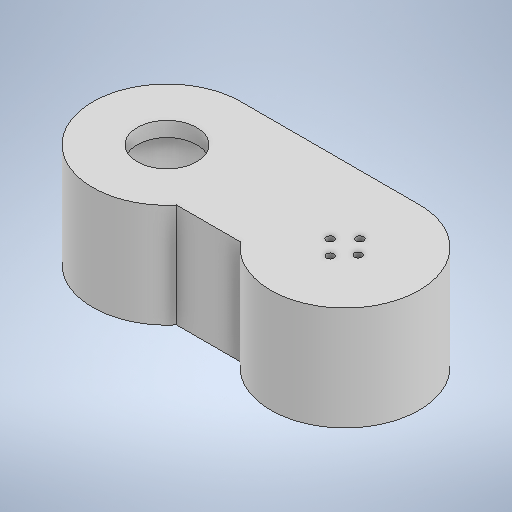
# Autodesk Inventor part: con_v6_d1
Saved by Autodesk Inventor 2025.4 (Build 294407000, 407)
## iProperties
Created: 2026-07-20
Part Number: con_v6_d1
Material: Generic
Document SubType Name: Modeling
Designer: Franchesca
Density: 1 g/cm^3
Appearance: Default
Author: Franchesca
## iProperties of the stored document con_v6_d1_3DPrint.ipt
Created: 2026-07-20
Part Number: con_v6_d1_3DPrint
Material: Generic
Document SubType Name: Modeling
Designer: Franchesca
Density: 1 g/cm^3
Appearance: Default
Author: Franchesca
Autodesk Inventor part; units mm, degrees
ref_plane "YZ Plane" through (0, 0, 0) normal (1, 0, 0) x (0, 1, 0)
sketch "Sketch1" plane through (0, 0, 0) normal (0, 1, 0) x (-1, 0, 0)
  line L0 (30, 0) -> (-30, 0) construction
  line L1 (30, 25) -> (-30, 25) construction
  line L2 (-30, -25) -> (30, -25)
  arc A0 (30, -25) -> (30, 25) centre (30, 0) ccw construction
  arc A1 (-30, 25) -> (-30, -25) centre (-30, 0) ccw
  line L3 (30, -25) -> (0, 0) construction
  line L4 (0, 0) -> (30, 25) construction
  line L5 (0, 0) -> (-34.4376, -24.603) construction
  line L6 (0, 0) -> (-34.4376, 25) construction
  line L7 (-34.4376, -24.603) -> (-34.4376, 25) construction
  line L8 (30, -25) -> (30, 25) construction
  line L9 (55, 0) -> (30, -25) construction
  line L10 (55, 0) -> (30, 25) construction
  line L11 (-34.4376, -24.603) -> (-55, 0) construction
  line L12 (-55, 0) -> (-30, 25) construction
  line L13 (25, 0) -> (-25, 0) construction
  line L14 (25, 25) -> (-25, 25) construction
  line L15 (-25, -25) -> (25, -25) construction
  arc A2 (25, -25) -> (25, 25) centre (25, 0) ccw construction
  arc A3 (-25, 25) -> (-25, -25) centre (-25, 0) ccw construction
  line L16 (55, 0) -> (25, -25) construction
  line L17 (55, 0) -> (25, 25) construction
  line L18 (25, -25) -> (25, 25) construction
  line L19 (0, 0) -> (55, 0) construction
  line L20 (-25, -25) -> (-25, 25) construction
  circle A4 centre (-30, 0) radius 25 construction
  circle A5 centre (30, 0) radius 25 construction
  circle A6 centre (-30, 0) radius 22.5 construction
  line L21 (30, -25) -> (-30, -25)
  line L22 (0, -25) -> (0, 25) construction
  line L23 (30, 0) -> (0, 25) construction
  line L24 (10.7945, 16.0046) -> (-10.7945, 16.0046) construction
  line L25 (10.7945, 16.0046) -> (-10.7945, 16.0046)
  line L26 (8.9613, 13.5046) -> (-8.9613, 13.5046)
  circle A7 centre (30, 0) radius 10
  line L27 (19.1028, -22.5) -> (-19.1028, -22.5)
  line L28 (-30, 0) -> (-30, -25) construction
  line L29 (-30, 0) -> (-30, 25) construction
  line L30 (-30, 0) -> (-12.3223, -17.6777) construction
  line L31 (-30, 0) -> (-47.6777, -17.6777) construction
  line L32 (-25, -5) -> (-34.4376, -5) construction
  line L33 (-12.3223, -17.6777) -> (-47.6777, 17.6777) construction
  line L34 (-47.6777, -17.6777) -> (-12.3223, 17.6777) construction
  line L35 (-25, 5) -> (-34.4376, 5) construction
  circle A8 centre (-30, -5) radius 1.25
  circle A9 centre (-25, 0) radius 1.25
  circle A10 centre (-34.4376, 0) radius 1.25
  circle A11 centre (-30, 5) radius 1.25
  line L36 (-19.1028, -22.5) -> (-19.1028, 22.5) construction
  line L37 (19.1028, -22.5) -> (19.0552, 22.4769) construction
  line L38 (10.7945, 16.0046) -> (10.7945, -22.5636) construction
  line L39 (10.7945, 16.0046) -> (49.3627, 16.0046) construction
  line L40 (-10.7945, 16.0046) -> (-10.7945, -22.0758) construction
  line L41 (-10.7945, 16.0046) -> (27.2859, 16.0046) construction
  line L42 (-10.7945, -22.0758) -> (-11.3044, -22.5) construction
  line L43 (-8.9613, 13.5046) -> (-8.9613, -22.5) construction
  line L44 (8.9613, 13.5046) -> (8.9613, -22.5) construction
  arc A12 (19.0998, -19.6834) -> (30, -22.5) centre (30, 0) ccw
  arc A13 (30, -22.5) -> (52.5, 0) centre (30, 0) ccw
  arc A14 (52.5, 0) -> (30, 22.5) centre (30, 0) ccw
  arc A15 (39.375, 20.4538) -> (19.0582, 19.6603) centre (30, 0) ccw
  circle A16 centre (30, 0) radius 22.5369 construction
  arc A17 (19.0582, 19.6603) -> (11.9574, 13.5046) centre (29.9457, -0.0723) ccw
  line L45 (8.9613, 13.5046) -> (11.9574, 13.5046)
  line L46 (19.0998, -19.6834) -> (19.1028, -22.5)
  arc A18 (30, 25) -> (10.7945, 16.0046) centre (30, 0) ccw
  arc A19 (55, 0) -> (30, 25) centre (30, 0) ccw
  arc A20 (30, -25) -> (55, 0) centre (30, 0) ccw
  arc A21 (-52.4985, -0.2589) -> (-19.1028, -19.685) centre (-30, 0) ccw
  arc A22 (-19.1028, 19.685) -> (-52.4985, -0.2589) centre (-30, 0) ccw
  line L47 (-8.9613, 13.5046) -> (-12.0035, 13.5046)
  arc A23 (-12.0035, 13.5046) -> (-19.1028, 19.685) centre (-30, 0) ccw
  line L48 (-19.1028, -22.5) -> (-19.1028, -19.685)
  arc A24 (-10.7945, 16.0046) -> (-30, 25) centre (-30, 0) ccw
  point P0 (-30, 25)
  point P1 (-30, 0)
  dimension "d1" = 30
  dimension "d2" = 50
  dimension "d3" = 50
  dimension "d4" = 25
  dimension "d8" = 110
  dimension "d9" = 50
  dimension "d12" = 45
  dimension "d13" = 0
  dimension "d14" = 2.5
  dimension "d15" = 20
  dimension "d16" = 2.5
  dimension "d25" = 2.5
  dimension "d26" = 2.5
  dimension "d27" = 2.5
  dimension "d28" = 2.5
  dimension "d29" = 90
  dimension "d30" = 90
  constraints: 102 end point, 50 point on circle, 28 point on line, 23 centre point, 9 perpendicular, 9 tangent, 7 coincident, 6 midpoint, 5 concentric, 5 horizontal, 4 collinear, 4 parallel, 3 vertical, 19 other
  measures "d1" distance of L3.end L0.end
  measures "d2" diameter of A1
  measures "d3" distance between parallel lines of L1 L2
  measures "d4" distance of L3.end L13.end
  measures "d8" distance of L11.end L9.start
  measures "d9" diameter of A5
  measures "d12" diameter of A6
  measures "d13" distance between parallel lines of L15 L2
  measures "d14" distance between parallel lines of L24 L26
  measures "d15" diameter of A7
  measures "d16" distance between parallel lines of L27 L15
  measures "d25" diameter of A8
  measures "d26" diameter of A9
  measures "d27" diameter of A10
  measures "d28" diameter of A11
  measures "d29" angle of L38 L39
  measures "d30" angle of L40 L41
ref_plane "Work Plane1" through (0, -5, 0) normal (0, -1, 0) x (1, 0, 0)
extrude "Extrusion2" add sketch "Sketch1" against normal blind 35 contours A1 A24 L25 A18 A19 A20 L2
extrude "Extrusion3" add sketch "Sketch1" against normal blind 5 contours L45 A17 A15 A14 A13 A12 L46 L27 L48 A21 A22 A23 L47 L26
sketch "Sketch3" plane through (0, -35, 0) normal (0, -1, 0) x (1, 0, 0)
  point P0 (0, 0)
ref_plane "Work Plane2" through (0, -35, 0) normal (0, -1, 0) x (1, 0, 0)
sketch "Sketch4" plane through (0, -35, 0) normal (0, -1, 0) x (1, 0, 0)
  line L0 (0, 0) -> (-55, 0) construction
  arc A0 (-10.7945, 16.0046) -> (-30, -25) centre (-30, 0) ccw construction
  arc A1 (30, -25) -> (10.7945, 16.0046) centre (30, 0) ccw construction
  line L1 (0, 0) -> (55, 0) construction
  line L2 (-30, -25) -> (-30, 25) construction
  line L3 (30, -25) -> (30, 25) construction
  line L4 (-30, 13.5046) -> (30, 13.5046) construction
  line L5 (-19.1028, -22.5) -> (-19.0998, -19.6834) construction
  line L6 (-19.0998, -19.6834) -> (-30, -19.6834) construction
  arc A2 (-19.0582, 19.6603) -> (-19.0998, -19.6834) centre (-30, 0) ccw construction
  line L7 (-19.0998, -19.6834) -> (30, -19.6834) construction
  circle A3 centre (-53.8, 0) radius 0.75
  circle A4 centre (53.8, 0) radius 0.75
  arc A5 (19.1028, -19.685) -> (12.0035, 13.5046) centre (30, 0) ccw construction
  line L8 (-10.7945, 16.0046) -> (-10.7945, 13.5046) construction
  line L9 (10.7945, 16.0046) -> (10.7945, 13.5046) construction
  circle A6 centre (-10.7945, 14.7546) radius 0.75
  circle A7 centre (10.7945, 14.7546) radius 0.75
  point P0 (-52.5, 0.0238)
  point P1 (-52.5, 0.0238)
  dimension "d41" = 2.5
  dimension "d42" = 1.5
  dimension "d43" = 1.3
  dimension "d44" = 1.5
  dimension "d45" = 0.55
  dimension "d46" = 1.5
  dimension "d47" = 1.5
  dimension "d48" = 20.0889
  constraints: 18 end point, 9 point on line, 6 point on circle, 5 perpendicular, 4 centre point, 2 horizontal, 2 midpoint, 1 parallel
  measures "d41" horizontal distance of L0.end point (-52.5, 0.024)
  measures "d42" diameter of A3
  measures "d43" horizontal distance of A3.centre point (-52.5, 0.024)
  measures "d44" diameter of A4
  measures "d46" diameter of A6
  measures "d47" diameter of A7
extrude "Extrusion4" cut sketch "Sketch4" against normal blind 5
body "Solid2"
